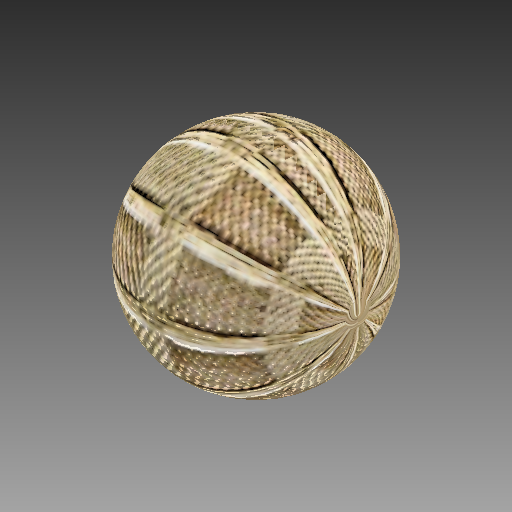
# Autodesk Inventor part: ball
Saved by Autodesk Inventor 2020 (Build 240168000, 168)
## iProperties
Created: 2024-09-28
Part Number: ball
Material: Типовые
Document SubType Name: Modeling
Designer: Ivan
Density: 1 g/cm^3
Appearance: Шотландка — бежевая
Mass: 212.175 g
Surface Area: 172.034 cm^2
Volume: 212.175 cm^3
Author: Ivan
Autodesk Inventor part; units mm, degrees
ref_plane "YZ Plane" through (0, 0, 0) normal (1, 0, 0) x (0, 1, 0)
ref_plane "XZ Plane" through (0, 0, 0) normal (0, 1, 0) x (-1, 0, 0)
ref_plane "XY Plane" through (0, 0, 0) normal (0, 0, 1) x (1, 0, 0)
sketch "Эскиз1" plane through (0, 0, 0) normal (0, 1, 0) x (-1, 0, 0)
  arc A0 (37, 0) -> (-37, 0) centre (0, 0) ccw
  line L0 (37, 0) -> (-37, 0)
  dimension "d0" = 37
  constraints: 2 end point, 2 point on circle, 1 centre point, 1 coincident, 1 horizontal
  measures "d0" radius of A0
revolve "Вращение1" add sketch "Эскиз1" angle 360 about axis through (-37, 0, 0) along (1, 0, 0)
